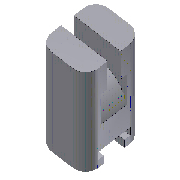
# Autodesk Inventor part: "ULC 1001"
Saved by Autodesk Inventor 2024 (Build 280153000, 153)
## iProperties
Created: 2023-01-19
Part Number: "ULC 1001"
Material: DIN 1.2344
Description: Coupling
Document SubType Name: Modeling
Designer: Alex
Standard Revision: 1
Manufacturer: DME
Language: en-US
Size Designation: "1001"
Categories: <MemberInstance><Categories><Category DisplayName="Mold" InternalName="349578f2-f4d4-4954-8c09-8e99297a61c0" Mnemonic="MOLD"><Category DisplayName="Lifter Components" InternalName="7bf15405-3151-40fb-a523-580ccd9f5458" Mnemonic="LIFTER COMPONENTS"><Category DisplayName="Couplings" InternalName="20259b59-cd45-429b-9f00-a2fc264bed37" Mnemonic="COUPLINGS"><CategoryParameter DisplayName="Trough Radius" InternalName="1b11b4e8-2d1a-403f-affc-fb5c003097d6" Mnemonic="TROUGH RADIUS"/><CategoryParameter DisplayName="Pin1 Distance" InternalName="2c0c3970-d07a-4fea-ac23-9049491c48c3" Mnemonic="PIN1 DISTANCE"/><CategoryParameter DisplayName="Hole Diameter" InternalName="496a63bf-b7a6-4788-bdf3-5a74f990b182" Mnemonic="HOLE DIAMETER"/><CategoryParameter DisplayName="Total Length" InternalName="56f84e39-1806-463a-ae91-d5a13db01532" Mnemonic="TOTAL LENGTH"/><CategoryParameter DisplayName="Angle" InternalName="6afdcf5e-a259-4143-aa1d-73cf01eddfb4" Mnemonic="ANGLE"/><CategoryParameter DisplayName="Shaft Diameter" InternalName="79037e71-a182-4bac-9451-726fb597494a" Mnemonic="SHAFT DIAMETER"/><CategoryParameter DisplayName="Hinge Pin Diameter" InternalName="97415974-4936-4bff-97fc-45fde78ed117" Mnemonic="HINGE PIN DIAMETER"/><CategoryParameter DisplayName="Total Height" InternalName="ba11b263-b03f-46e7-8623-a5a29b421ba8" Mnemonic="TOTAL HEIGHT"/><CategoryParameter DisplayName="Total Width" InternalName="dd899064-5edc-47be-b52f-13e871c69d5c" Mnemonic="TOTAL WIDTH"/></Category></Category></Category><Category DisplayName="DataType" InternalName="23b78d0f-2648-40c6-8793-ca6db495c9e8" Mnemonic="DATATYPE"><CategoryParameter DisplayName="DisplayName" InternalName="05415f3d-3907-474b-a020-eb9d644f4cf3" Mnemonic="DISPLAYNAME"/><CategoryParameter DisplayName="Standard" InternalName="0c0a119c-1e12-4c84-803f-101930972f5e" Mnemonic="STANDARD"/><CategoryParameter DisplayName="Description" InternalName="13903e3d-64b1-4950-80da-f627842ea37f" Mnemonic="DESCRIPTION"/><CategoryParameter DisplayName="Designation" InternalName="2675968c-4ce5-49e0-a4f5-552d29089031" Mnemonic="DESIGNATION"/><CategoryParameter DisplayName="Default Row" InternalName="2af9ec52-faaa-4026-b378-f9fa4afca842" Mnemonic="DEFAULTROW"/><CategoryParameter DisplayName="Folder Name" InternalName="3f06958e-8713-4116-9be7-ed6184ecc97b" Mnemonic="FOLDERNAME"/><CategoryParameter DisplayName="Revision Guid" InternalName="45a75005-10b1-4dfc-8d6d-dfe629f0b93c" Mnemonic="REVISIONGUID"/><CategoryParameter DisplayName="FileName" InternalName="8b46a4cc-9585-4fed-90c3-899f57e09a73" Mnemonic="FILENAME"/><CategoryParameter DisplayName="StdsOrg" InternalName="8f5914e1-4693-403f-8ab5-d37768198c9d" Mnemonic="STDSORG"/><CategoryParameter DisplayName="Family Version" InternalName="914462f6-6e19-4b14-ba84-155b9680b1d0" Mnemonic="FAMILYREVISION"/><CategoryParameter DisplayName="Standard Revision" InternalName="91d5a463-65c2-4fde-b823-3b7fea5e8e17" Mnemonic="STANDARDREVISION"/><CategoryParameter DisplayName="Member Revision" InternalName="a65d44b9-392f-4f4f-857b-e4b3d54996fe" Mnemonic="MEMBERREVISION"/><CategoryParameter DisplayName="ClipFormat" InternalName="bc51e27b-3422-4e78-93ef-cec197ddf230" Mnemonic="CLIPFORMAT"/><CategoryParameter DisplayName="Manufacturer" InternalName="cd6c7a72-a28a-4e50-99a9-2c7f4e13e5ad" Mnemonic="MANUFACTURER"/><CategoryParameter DisplayName="InternalName" InternalName="cf1d0246-76d9-4b4a-8305-fa0409afb5c1" Mnemonic="INTERNALNAME"/><CategoryParameter DisplayName="IsMetric" InternalName="e2385c5b-1ea4-4823-96a8-8de651266ec3" Mnemonic="ISMETRIC"/><Category DisplayName="Part" InternalName="c0e0b642-3bcb-4cc8-9e80-f96d35c4afa4" Mnemonic="PART"><CategoryParameter DisplayName="Part Number" InternalName="016b6077-bfbe-49bd-92c9-d8d59c39c941" Mnemonic="PARTNUMBER"/><CategoryParameter DisplayName="Stock Number" InternalName="4dba7c1c-e26c-444e-836c-b08b433409a8" Mnemonic="STOCKNUMBER"/><CategoryParameter DisplayName="Material Key" InternalName="5c9a8adb-dd2b-4535-b97f-0a94a95fe41f" Mnemonic="MATERIALKEY"/><CategoryParameter DisplayName="Material" InternalName="818a152a-d3c3-49ca-80ee-df7d91421b8e" Mnemonic="MATERIAL"/></Category></Category></Categories><FamilyTemplate Id="ULC"><FamilyTemplateParameters><FamilyTemplateParameter ObjectType="kUserParameterObject" ValueType="xs:double" Id="1" ObjectReferenceKey="W_"/><FamilyTemplateParameter ObjectType="kUserParameterObject" ValueType="xs:double" Id="2" ObjectReferenceKey="L"/><FamilyTemplateParameter ObjectType="kUserParameterObject" ValueType="xs:double" Id="3" ObjectReferenceKey="H_"/><FamilyTemplateParameter ObjectType="kUserParameterObject" ValueType="xs:double" Id="4" ObjectReferenceKey="ULC_ULB_H"/><FamilyTemplateParameter ObjectType="kUserParameterObject" ValueType="xs:double" Id="5" ObjectReferenceKey="RC"/><FamilyTemplateParameter ObjectType="kUserParameterObject" ValueType="xs:double" Id="6" ObjectReferenceKey="R"/><FamilyTemplateParameter ObjectType="kUserParameterObject" ValueType="xs:double" Id="7" ObjectReferenceKey="ULC_ULB_Wmin"/><FamilyTemplateParameter ObjectType="kUserParameterObject" ValueType="xs:double" Id="8" ObjectReferenceKey="ULC_ULB_W1"/><FamilyTemplateParameter ObjectType="kUserParameterObject" ValueType="xs:double" Id="9" ObjectReferenceKey="ULC_ULG_W1"/><FamilyTemplateParameter ObjectType="kUserParameterObject" ValueType="xs:double" Id="10" ObjectReferenceKey="ULC_ULG_W2"/><FamilyTemplateParameter ObjectType="kUserParameterObject" ValueType="xs:double" Id="11" ObjectReferenceKey="ULC_ULG_H1"/><FamilyTemplateParameter ObjectType="kUserParameterObject" ValueType="xs:double" Id="12" ObjectReferenceKey="ULC_ULG_H2"/><FamilyTemplateParameter ObjectType="kPartComponentDefinitionObject" ValueType="xs:string" Id="13" SubObjectId="Material"/><FamilyTemplateParameter ObjectType="kPropertyObject" ValueType="xs:string" Id="22" ObjectReferenceKey="{32853F0F-3444-11d1-9E93-0060B03C1CA6}" SubObjectId="5"/><FamilyTemplateParameter ObjectType="kPropertyObject" ValueType="xs:string" Id="23" ObjectReferenceKey="{32853F0F-3444-11d1-9E93-0060B03C1CA6}" SubObjectId="52"/></FamilyTemplateParameters></FamilyTemplate><CategoryParameterMap><ParamToTemplateMap><ParamToTemplate CategoryParameter="//CategoryParameter[@InternalName='2af9ec52-faaa-4026-b378-f9fa4afca842']" ConstantValue="1"/><ParamToTemplate CategoryParameter="//CategoryParameter[@InternalName='bc51e27b-3422-4e78-93ef-cec197ddf230']" ConstantValue="CF_INVENTOR.STDPARTS"/><ParamToTemplate CategoryParameter="//CategoryParameter[@InternalName='e2385c5b-1ea4-4823-96a8-8de651266ec3']" ConstantValue="true"/><ParamToTemplate CategoryParameter="//CategoryParameter[@InternalName='cf1d0246-76d9-4b4a-8305-fa0409afb5c1']" ConstantValue="492e7e86-02dd-4aaa-8f6c-7f27e3159fab"/><ParamToTemplate CategoryParameter="//CategoryParameter[@InternalName='45a75005-10b1-4dfc-8d6d-dfe629f0b93c']" ConstantValue="175dd14f-d69c-4763-b006-9ceafa53336a"/><ParamToTemplate CategoryParameter="//CategoryParameter[@InternalName='3f06958e-8713-4116-9be7-ed6184ecc97b']" ConstantValue="ULC"/><ParamToTemplate CategoryParameter="//CategoryParameter[@InternalName='8f5914e1-4693-403f-8ab5-d37768198c9d']" TemplateParameter="17"/><ParamToTemplate CategoryParameter="//CategoryParameter[@InternalName='0c0a119c-1e12-4c84-803f-101930972f5e']" TemplateParameter="18"/><ParamToTemplate CategoryParameter="//CategoryParameter[@InternalName='91d5a463-65c2-4fde-b823-3b7fea5e8e17']" ConstantValue="1"/><ParamToTemplate CategoryParameter="//CategoryParameter[@InternalName='cd6c7a72-a28a-4e50-99a9-2c7f4e13e5ad']" ConstantValue="DME"/><ParamToTemplate CategoryParameter="//CategoryParameter[@InternalName='13903e3d-64b1-4950-80da-f627842ea37f']" ConstantValue="Coupling"/><ParamToTemplate CategoryParameter="//CategoryParameter[@InternalName='05415f3d-3907-474b-a020-eb9d644f4cf3']" ConstantValue="ULC"/><ParamToTemplate CategoryParameter="//CategoryParameter[@InternalName='914462f6-6e19-4b14-ba84-155b9680b1d0']" ConstantValue="1"/><ParamToTemplate CategoryParameter="//CategoryParameter[@InternalName='bc51e27b-3422-4e78-93ef-cec197ddf230']" ConstantValue="CF_INVENTOR.STDPARTS"/><ParamToTemplate CategoryParameter="//CategoryParameter[@InternalName='8b46a4cc-9585-4fed-90c3-899f57e09a73']" ConstantValue="&quot;ULC 1001&quot;"/><ParamToTemplate CategoryParameter="//CategoryParameter[@InternalName='a65d44b9-392f-4f4f-857b-e4b3d54996fe']" ConstantValue="E78DBA38-7AF7-4A6E-8A36-50846AAB9521"/><ParamToTemplate CategoryParameter="//CategoryParameter[@InternalName='2675968c-4ce5-49e0-a4f5-552d29089031']" TemplateParameter="23"/><ParamToTemplate CategoryParameter="//CategoryParameter[@InternalName='ba11b263-b03f-46e7-8623-a5a29b421ba8']" TemplateParameter="3"/><ParamToTemplate CategoryParameter="//CategoryParameter[@InternalName='56f84e39-1806-463a-ae91-d5a13db01532']" TemplateParameter="2"/><ParamToTemplate CategoryParameter="//CategoryParameter[@InternalName='818a152a-d3c3-49ca-80ee-df7d91421b8e']" TemplateParameter="13"/><ParamToTemplate CategoryParameter="//CategoryParameter[@InternalName='016b6077-bfbe-49bd-92c9-d8d59c39c941']" TemplateParameter="22"/><ParamToTemplate CategoryParameter="//CategoryParameter[@InternalName='1b11b4e8-2d1a-403f-affc-fb5c003097d6']" TemplateParameter="6"/><ParamToTemplate CategoryParameter="//CategoryParameter[@InternalName='dd899064-5edc-47be-b52f-13e871c69d5c']" TemplateParameter="1"/></ParamToTemplateMap></CategoryParameterMap></MemberInstance>
Density: 25 g/cm^3
Appearance: Smooth - Dark Sea Green
IsCustomPart: 1
Author: Alex
Autodesk Inventor part; units mm, degrees
ref_plane "YZ Plane" through (0, 0, 0) normal (1, 0, 0) x (0, 1, 0)
ref_plane "XZ Plane" through (0, 0, 0) normal (0, 1, 0) x (-1, 0, 0)
sketch "Sketch1" plane through (0, 0, 0) normal (1, 0, 0) x (0, 1, 0)
  line L0 (0, -9) -> (0, 26) projected
  line L1 (0, 21) -> (-11, 21)
  line L2 (-11, 21) -> (-11, -4)
  line L3 (-11, -4) -> (-4, -4)
  line L4 (-4, -4) -> (-4, -2)
  line L5 (-4, -2) -> (-6.25, -2)
  line L6 (-6.25, -2) -> (-6.25, 0)
  line L7 (-6.25, 0) -> (0, 0)
  line L8 (0, 21) -> (11, 21)
  line L9 (11, 21) -> (11, -4)
  line L10 (11, -4) -> (4, -4)
  line L11 (4, -4) -> (4, -2)
  line L12 (4, -2) -> (6.25, -2)
  line L13 (6.25, -2) -> (6.25, 0)
  line L14 (6.25, 0) -> (0, 0)
  dimension "d1" = 22
  dimension "d2" = 25
  dimension "d3" = 12.5
  dimension "d4" = 8
  dimension "d5" = 4
  dimension "d6" = 2
  constraints: 28 end point, 6 symmetric about line, 4 perpendicular, 3 parallel, 1 horizontal, 1 point on line
  measures "d1" diameter of L2 L0
  measures "d2" distance between parallel lines of L3 L1
  measures "d3" diameter of L6 L0
  measures "d4" diameter of L4 L0
  measures "d5" distance between parallel lines of L3 L7
  measures "d6" distance between parallel lines of L3 L5
extrude "Extrusion1" add sketch "Sketch1" along normal blind 18
fillet "Fillet1" radius 5 4 edges at (0, -11, 8.5) (18, -11, 8.5) (18, 11, 8.5) (0, 11, 8.5)
sketch "Sketch2" plane through (0, 0, 0) normal (0, 1, 0) x (-1, 0, 0)
  line L0 (-18, 0) -> (-18, 21) construction
  line L1 (-5, 21) -> (-13, 21) construction
  line L2 (-9, 21) -> (-9, -4)
  line L3 (0, -4) -> (-18, -4) construction
  line L4 (0, 0) -> (0, 0) construction
  arc A0 (0, 6.3589) -> (-18, 6.3589) centre (-9, 2) ccw
  arc A1 (0, 14) -> (-18, 14) centre (-9, 2) ccw
  line L5 (-18, 14) -> (-18, 6.3589)
  line L6 (0, 6.3589) -> (0, 14)
  line L7 (0, 14) -> (0, 6.3589)
  line L8 (-18, 14) -> (-18, 21)
  line L9 (-18, 21) -> (0, 21)
  line L10 (0, 21) -> (0, 14)
  dimension "d10" = 10
  dimension "d11" = 6
  dimension "d18" = 5
  constraints: 14 end point, 5 point on line, 4 collinear, 4 point on circle, 2 centre point, 2 midpoint, 2 perpendicular, 1 coincident
  measures "d10" radius of A0
  measures "d11" distance of L2.end A0.centre
  measures "d18" radial gap between concentric circles of A0 A1
extrude "Extrusion2" cut sketch "Sketch2" against normal mid plane 10 contours A1 L6 A0 L2 | L2 A0 L5 A1
extrude "Extrusion3" cut sketch "Sketch2" against normal mid plane 5 contours L9 L10 A1 L2 | L2 A1 L8 L9
ref_plane "ULC_ULG" through (18, 0, 0) normal (1, 0, 0) x (0, 0, -1)
equation "\"d1\" = W_"
equation "\"d2\" = H_"
equation "\"d3\" = ULC_ULG_W1"
equation "\"d4\" = ULC_ULG_W2"
equation "\"d5\" = ULC_ULG_H1"
equation "\"d6\" = ULC_ULG_H2"
equation "\"d7\" = L"
equation "\"d9\" = ULC_a1"
equation "\"d10\" = R"
equation "\"d11\" = RC"
equation "\"d18\" = ULC_ULB_H"
equation "\"d19\" = ULC_ULB_Wmin"
equation "\"d23\" = ULC_ULB_W1"
equation "\"ULC_ULB_H\" = 5"
equation "\"W_\" = 22"
equation "\"L\" = 18"
equation "\"H_\" = 25"
equation "\"RC\" = 6"
equation "\"R\" = 10"
equation "\"ULC_ULB_Wmin\" = 10"
equation "\"ULC_ULB_W1\" = 5"
equation "\"ULC_ULG_W1\" = 12.5"
equation "\"ULC_ULG_W2\" = 8"
equation "\"ULC_ULG_H1\" = 4"
equation "\"ULC_ULG_H2\" = 2"
equation "\"ULC_a1\" = 5"
body "Solid1"
